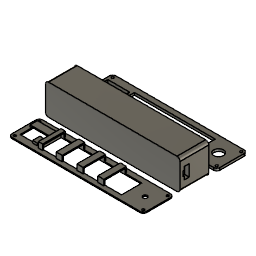
pomodoro (Autodesk Fusion 360 design; units mm, degrees)
Autodesk Fusion 360 part; units mm, degrees
sketch "Sketch1" plane through (0, 0, 0) normal (0, 0, 1) x (1, 0, 0)
  line L0 (66, 16.5) -> (-66, 16.5)
  line L1 (-66, 16.5) -> (-66, -16.5)
  line L2 (-66, -16.5) -> (66, -16.5)
  line L3 (66, -16.5) -> (66, 16.5)
  line L4 (66, 16.5) -> (-66, -16.5) construction
  line L5 (-66, 16.5) -> (66, -16.5) construction
  circle A0 centre (88, 0) radius 3.5
  line L6 (-74, 14) -> (-102, 14)
  line L7 (-102, 14) -> (-102, -14)
  line L8 (-102, -14) -> (-74, -14)
  line L9 (-74, -14) -> (-74, 14)
  line L10 (-74, 14) -> (-102, -14) construction
  line L11 (-102, 14) -> (-74, -14) construction
  line L12 (105, 25) -> (-105, 25)
  line L13 (-110, 20) -> (-110, -20)
  line L14 (-105, -25) -> (105, -25)
  line L15 (110, -20) -> (110, 20)
  line L16 (110, 25) -> (-110, -25) construction
  line L17 (-110, 25) -> (110, -25) construction
  circle A1 centre (88, 0) radius 8
  line L18 (-74, 9) -> (-102, 9)
  line L19 (-102, 9) -> (-102, -6)
  line L20 (-102, -6) -> (-74, -6)
  line L21 (-74, -6) -> (-74, 9)
  arc A2 (110, 20) -> (105, 25) centre (105, 20) ccw
  arc A3 (105, -25) -> (110, -20) centre (105, -20) ccw
  arc A4 (-110, -20) -> (-105, -25) centre (-105, -20) ccw
  arc A5 (-105, 25) -> (-110, 20) centre (-105, 20) ccw
  circle A6 centre (-105, -20) radius 2
  circle A7 centre (-105, 20) radius 2
  circle A8 centre (105, 20) radius 2
  circle A9 centre (105, -20) radius 2
  line L22 (-68, 18.5) -> (-61, 18.5)
  line L23 (-61, 18.5) -> (-61, -18.5)
  line L24 (-61, -18.5) -> (-68, -18.5)
  line L25 (-68, -18.5) -> (-68, 18.5)
  line L26 (-39, 18.5) -> (-29, 18.5)
  line L27 (-29, 18.5) -> (-29, -18.5)
  line L28 (-29, -18.5) -> (-39, -18.5)
  line L29 (-39, -18.5) -> (-39, 18.5)
  line L30 (-5, 18.5) -> (5, 18.5)
  line L31 (5, 18.5) -> (5, -18.5)
  line L32 (5, -18.5) -> (-5, -18.5)
  line L33 (-5, -18.5) -> (-5, 18.5)
  line L34 (0, 2.5) -> (0, 20)
  line L35 (39, 18.5) -> (29, 18.5)
  line L36 (29, 18.5) -> (29, -18.5)
  line L37 (29, -18.5) -> (39, -18.5)
  line L38 (39, -18.5) -> (39, 18.5)
  line L39 (-72, -16) -> (-104, -16)
  line L40 (-104, -16) -> (-104, -4)
  line L41 (-104, -4) -> (-72, -4)
  line L42 (-72, -4) -> (-72, -16)
  line L43 (-72, 16) -> (-80, 16)
  line L44 (-80, 16) -> (-80, 4)
  line L45 (-80, 4) -> (-72, 4)
  line L46 (-72, 4) -> (-72, 16)
  point P0 (-88, 0)
  dimension "d1" = 132
  dimension "d2" = 33
  dimension "d4" = 7
  dimension "d5" = 28
  dimension "d6" = 28
  dimension "d7" = 22
  dimension "d8" = 22
  dimension "d9" = 220
  dimension "d10" = 50
  dimension "d11" = 16
  dimension "d12" = 5
  dimension "d13" = 15
  dimension "d14" = 5
  dimension "d15" = 4
  dimension "d16" = 4
  dimension "d17" = 4
  dimension "d18" = 4
  dimension "d59" = 7
  dimension "d60" = 37
  dimension "d61" = 10
  dimension "d62" = 37
  dimension "d63" = 27
  dimension "d64" = 37
  dimension "d65" = 61
  constraint horizontal L0
  constraint perpendicular L0 L1
  constraint parallel L0 L2
  constraint parallel L1 L3
  constraint coincident L4 origin
  constraint coincident L5 origin
  constraint horizontal L6
  constraint perpendicular L6 L7
  constraint parallel L6 L8
  constraint parallel L7 L9
  constraint coincident L10 P0
  constraint coincident L11 P0
  constraint horizontal L12
  constraint perpendicular L12 L13
  constraint parallel L12 L14
  constraint parallel L13 L15
  constraint coincident L16 origin
  constraint coincident L17 origin
  constraint concentric A0 A1
  constraint horizontal L18
  constraint vertical L19
  constraint horizontal L20
  constraint vertical L21
  constraint coincident L7 L19.end
  constraint coincident L9 L18.start
  constraint coincident L16.start L12
  constraint coincident L16.start L15
  constraint tangent L12 A2
  constraint tangent L15 A2
  constraint coincident L17.end L15
  constraint coincident L17.end L14
  constraint tangent L15 A3
  constraint tangent L14 A3
  constraint equal A2 A3
  constraint coincident L16.end L13
  constraint coincident L16.end L14
  constraint tangent L13 A4
  constraint tangent L14 A4
  constraint equal A2 A4
  constraint coincident L17.start L12
  constraint coincident L17.start L13
  constraint tangent L12 A5
  constraint tangent L13 A5
  constraint equal A2 A5
  constraint concentric A4 A6
  constraint concentric A5 A7
  constraint concentric A2 A8
  constraint concentric A3 A9
  constraint horizontal L22
  constraint vertical L23
  constraint horizontal L24
  constraint vertical L25
  constraint horizontal L26
  constraint vertical L27
  constraint horizontal L28
  constraint vertical L29
  constraint horizontal L30
  constraint vertical L31
  constraint horizontal L32
  constraint vertical L33
  constraint symmetric L26.start L34 L35.start
  constraint symmetric L26.end L34 L35.end
  constraint symmetric L27.end L34 L36.end
  constraint symmetric L28.end L34 L37.end
  constraint horizontal L39
  constraint vertical L40
  constraint horizontal L41
  constraint vertical L42
  constraint horizontal L43
  constraint vertical L44
  constraint horizontal L45
  constraint vertical L46
  measures "d1" distance of L1.end L2.end
  measures "d2" distance of L0.end L1.end
  measures "d4" diameter of A0
  measures "d5" distance of L7.end L8.end
  measures "d6" distance of L6.end L7.end
  measures "d7" distance of L1 P0
  measures "d8" distance of L3 A0.centre
  measures "d9" distance of L16.end L17.end
  measures "d10" distance of L17.start L16.end
  measures "d11" diameter of A1
  measures "d12" distance of L6 L18
  measures "d13" distance of L18 L20
  measures "d14" radius of A2
  measures "d15" diameter of A6
  measures "d16" diameter of A7
  measures "d17" diameter of A8
  measures "d18" diameter of A9
  measures "d59" distance of L22.start L22.end
  measures "d60" distance of L22.start L24.end
  measures "d61" distance of L26.start L26.end
  measures "d62" distance of L26.start L28.end
  measures "d63" distance of L1 L29
  measures "d64" distance of L30.start L32.end
  measures "d65" distance of L1 L33
extrude "Extrude1" add sketch "Sketch1" along normal blind 4 contours L0 L35 L36 L38 | L2 L36 L37 L38 | L0 L30 L31 L34 | L0 L30 L33 L34 | L2 L31 L32 L33 | L0 L26 L27 L29 | L2 L27 L28 L29 | L0 L1 L2 L22 L23 L24 L25 | L6 L9 L18 L44 | L6 L9 L21 L43 L44 L45 L46 | L6 L7 L18 L44 | L7 L8 L9 L19 L21 L39 L40 L41 L42 | L7 L8 L9 L20 | L12 L13 L14 L15 A2 A3 A4 A5 makes body 1
extrude "Extrude2" add sketch "Sketch1" against normal blind 1.8 separate body contours L0 L35 L36 L38 | L2 L36 L37 L38 | L0 L30 L31 L34 | L0 L30 L33 L34 | L2 L31 L32 L33 | L0 L26 L27 L29 | L2 L27 L28 L29 | L0 L1 L2 L22 L23 L24 L25 | L6 L9 L21 L43 L44 L45 L46 | L7 L8 L9 L19 L21 L39 L40 L41 L42 | L12 L13 L14 L15 A2 A3 A4 A5 | A1 makes body 2
move_body "Move1" bodies 1 to x (1, 0, 0) y (0, 1, 0) z (0, 0, 1) at (0, 60, 0)
extrude "Extrude13" add sketch "Sketch1" against normal blind 11 contours L0 L2 L36 L38 | L0 L35 L36 L38 | L2 L36 L37 L38 | L0 L2 L31 L33 | L0 L30 L31 L34 | L0 L30 L33 L34 | L2 L31 L32 L33 | L0 L2 L27 L29 | L0 L26 L27 L29 | L2 L27 L28 L29 | L0 L1 L2 L23 | L0 L1 L2 L22 L23 L24 L25 bodies 2
extrude "Extrude14" cut sketch "Sketch1" against normal blind 9 contours L0 L2 L36 L38 | L0 L2 L31 L33 | L0 L2 L27 L29 | L0 L1 L2 L23 bodies 2
extrude "Extrude15" add sketch "Sketch1" against normal blind 5.5 contours L6 L9 L18 L44 | L6 L9 L21 L43 L44 L45 L46 | L9 L18 L21 L44 L45 | L7 L8 L9 L19 L21 L39 L40 L41 L42 | L7 L9 L19 L20 L21 L41 | L7 L8 L9 L20 bodies 2
extrude "Extrude16" cut sketch "Sketch1" against normal blind 3.5 contours L6 L9 L18 L44 | L9 L18 L21 L44 L45 | L7 L9 L19 L20 L21 L41 | L7 L8 L9 L20 bodies 2
move_body "Move2" bodies 2 to x (1, 0, 0) y (0, 1, 0) z (0, 0, 1) at (0, 0, 1.8)
chamfer "Chamfer1" distance 4 distance2 3 4 edges at (-88, 69, 4) (-102, 61.5, 4) (-88, 54, 4) (-74, 61.5, 4) measured on face at (105.3333, 60, 4) measured on face at (105.3333, 60, 4) measured on face at (105.3333, 60, 4) measured on face at (105.3333, 60, 4) on bodies 1
sketch "Sketch2" plane through (0, 0, 0) normal (0, 0, 1) x (1, 0, 0)
  line L0 (-105, 25) -> (105, 25)
  line L1 (110, 20) -> (110, -20)
  line L2 (105, -25) -> (-105, -25)
  line L3 (-110, -20) -> (-110, 20)
  arc A0 (-105, 25) -> (-110, 20) centre (-105, 20) ccw
  arc A1 (-110, -20) -> (-105, -25) centre (-105, -20) ccw
  arc A2 (105, -25) -> (110, -20) centre (105, -20) ccw
  arc A3 (110, 20) -> (105, 25) centre (105, 20) ccw
  line L4 (-102.5, 17.5) -> (102.5, 17.5)
  line L5 (102.5, 17.5) -> (102.5, -17.5)
  line L6 (102.5, -17.5) -> (-102.5, -17.5)
  line L7 (-102.5, -17.5) -> (-102.5, 17.5)
  line L8 (110, -10) -> (65, -10)
  line L9 (65, -10) -> (65, 10)
  line L10 (65, 10) -> (110, 10)
  line L11 (110, 10) -> (110, -10)
  line L12 (65, -10) -> (102.5, -10)
  line L13 (102.5, -10) -> (102.5, -12)
  line L14 (102.5, -12) -> (65, -12)
  line L15 (65, -12) -> (65, -10)
  line L16 (65, 10) -> (102.5, 10)
  line L17 (102.5, 10) -> (102.5, 12)
  line L18 (102.5, 12) -> (65, 12)
  line L19 (65, 12) -> (65, 10)
  line L20 (65, -12) -> (63, -12)
  line L21 (63, -12) -> (63, -7)
  line L22 (63, -7) -> (65, -7)
  line L23 (65, -7) -> (65, -12)
  line L24 (65, 12) -> (63, 12)
  line L25 (63, 12) -> (63, 7)
  line L26 (63, 7) -> (65, 7)
  line L27 (65, 7) -> (65, 12)
  circle A4 centre (105, 20) radius 1
  circle A5 centre (105, -20) radius 1
  circle A6 centre (-105, -20) radius 1
  circle A7 centre (-105, 20) radius 1
  line L28 (-68.5, 19) -> (-60.5, 19)
  line L29 (-60.5, 19) -> (-60.5, -19)
  line L30 (-60.5, -19) -> (-68.5, -19)
  line L31 (-68.5, -19) -> (-68.5, 19)
  line L32 (-39.5, 19) -> (-28.5, 19)
  line L33 (-28.5, 19) -> (-28.5, -19)
  line L34 (-28.5, -19) -> (-39.5, -19)
  line L35 (-39.5, -19) -> (-39.5, 19)
  line L36 (-5.5, -19) -> (5.5, -19)
  line L37 (5.5, -19) -> (5.5, 19)
  line L38 (5.5, 19) -> (-5.5, 19)
  line L39 (-5.5, 19) -> (-5.5, -19)
  line L40 (28.5, 19) -> (39.5, 19)
  line L41 (39.5, 19) -> (39.5, -19)
  line L42 (39.5, -19) -> (28.5, -19)
  line L43 (28.5, -19) -> (28.5, 19)
  line L44 (-102.5, -16.5) -> (-105, -16.5)
  line L45 (-105, -16.5) -> (-105, -3.5)
  line L46 (-105, -3.5) -> (-102.5, -3.5)
  line L47 (-102.5, -3.5) -> (-102.5, -16.5)
  dimension "d25" = 5
  dimension "d46" = 45
  dimension "d47" = 20
  dimension "d48" = 2
  dimension "d49" = 2
  dimension "d50" = 2
  constraint horizontal L0
  constraint vertical L1
  constraint horizontal L2
  constraint vertical L3
  constraint tangent L0 A0
  constraint tangent L3 A0
  constraint tangent L2 A1
  constraint tangent L3 A1
  constraint equal A0 A1
  constraint tangent L1 A2
  constraint tangent L2 A2
  constraint equal A0 A2
  constraint tangent L0 A3
  constraint tangent L1 A3
  constraint equal A0 A3
  constraint horizontal L4
  constraint vertical L5
  constraint horizontal L6
  constraint vertical L7
  constraint horizontal L8
  constraint vertical L9
  constraint horizontal L10
  constraint vertical L11
  constraint coincident L1 L8.start
  constraint horizontal L12
  constraint vertical L13
  constraint horizontal L14
  constraint vertical L15
  constraint horizontal L16
  constraint vertical L17
  constraint horizontal L18
  constraint vertical L19
  constraint horizontal L20
  constraint vertical L21
  constraint horizontal L22
  constraint vertical L23
  constraint horizontal L24
  constraint vertical L25
  constraint horizontal L26
  constraint vertical L27
  constraint concentric A3 A4
  constraint concentric A2 A5
  constraint concentric A1 A6
  constraint concentric A0 A7
  constraint horizontal L28
  constraint vertical L29
  constraint horizontal L30
  constraint vertical L31
  constraint horizontal L32
  constraint vertical L33
  constraint horizontal L34
  constraint vertical L35
  constraint horizontal L36
  constraint vertical L37
  constraint horizontal L38
  constraint vertical L39
  constraint horizontal L40
  constraint vertical L41
  constraint horizontal L42
  constraint vertical L43
  constraint horizontal L44
  constraint vertical L45
  constraint horizontal L46
  constraint vertical L47
  constraint coincident L7 L44.start
  measures "d25" radius of A0
  measures "d46" distance of L8.start L8.end
  measures "d47" distance of L8.start L10.end
  measures "d48" distance of L8.end L14.end
  measures "d49" distance of L9.end L18.end
  measures "d50" distance of L14.end L20.end
extrude "Extrude3" add sketch "Sketch2" along normal blind 40 separate body contours L0 L1 L2 L3 A0 A1 A2 A3 L4 L5 L6 L7 L8 L10 L13 L17 L28 L29 L30 L31 L32 L33 L34 L35 L36 L37 L38 L39 L40 L41 L42 L43 L44 L45 L46 | L1 L5 L8 L10 L11 makes body 3
extrude "Extrude17" add sketch "Sketch2" along normal blind 30.5 contours L4 L40 L41 L43 | L6 L41 L42 L43 | L4 L37 L38 L39 | L6 L36 L37 L39 | L4 L32 L33 L35 | L6 L33 L34 L35 | L4 L28 L29 L31 | L6 L29 L30 L31 | L7 L44 L45 L46 L47 bodies 3
extrude "Extrude12" add sketch "Sketch2" along normal blind 39 contours A4 | A5 | A6 | A7 bodies 3
chamfer "Chamfer2" distance 1 distance2 0.7 4 edges at (-105.9323, 20.3616, 39) (-105.9323, -19.6384, 39) (104.0677, -19.6384, 39) (104.0677, 20.3616, 39) measured on face at (-104.4163, 20.8119, 39.3333) measured on face at (-104.6815, -19.0521, 39.3333) measured on face at (105.4113, -19.0885, 39.6667) measured on face at (105.4113, 20.9115, 39.6667) on bodies 3
move_body "Move3" bodies 2 to x (1, 0, 0) y (0, -1, 0) z (0, 0, -1) at (0, -60, 1.8)
extrude "Extrude4" add sketch "Sketch2" against normal blind 5 contours L0 L1 L2 L3 A0 A1 A2 A3 L4 L5 L6 L7 L8 L10 L13 L17 L28 L29 L30 L31 L32 L33 L34 L35 L36 L37 L38 L39 L40 L41 L42 L43 L44 L45 L46 | L1 L5 L8 L10 L11 | L5 L10 L16 L17 L18 L19 L27 | L5 L8 L9 L10 L12 L16 L23 L27 | L5 L8 L12 L13 L14 L15 L23 | L4 L5 L6 L9 L14 L18 L20 L21 L22 L24 L25 L26 L41 | L9 L19 L24 L25 L26 L27 | L9 L15 L20 L21 L22 L23 | L4 L6 L41 L43 | L4 L40 L41 L43 | L6 L41 L42 L43 | L4 L6 L37 L43 | L4 L6 L37 L39 | L4 L37 L38 L39 | L6 L36 L37 L39 | L4 L6 L33 L39 | L4 L6 L33 L35 | L4 L32 L33 L35 | L6 L33 L34 L35 | L4 L6 L29 L35 | L4 L6 L29 L31 | L4 L28 L29 L31 | L6 L29 L30 L31 | L4 L6 L7 L31 L47 | L7 L44 L45 L46 L47 | A4 | A5 | A6 | A7 bodies 3
sketch "Sketch3" plane through (110, 0, 0) normal (1, 0, 0) x (0, 1, 0)
  line L0 (20, -5) -> (20, 40)
  line L1 (20, 40) -> (-20, 40)
  line L2 (-20, 40) -> (-20, -5)
  line L3 (-20, -5) -> (20, -5)
  line L4 (-9.5, 0) -> (-9.5, 8)
  line L5 (-9.5, 8) -> (9.5, 8)
  line L6 (9.5, 8) -> (9.5, 0)
  line L7 (9.5, 0) -> (-9.5, 0)
  line L8 (4, -2) -> (-4, -2)
  line L9 (-4, -2) -> (-4, 2)
  line L10 (-4, 2) -> (4, 2)
  line L11 (4, 2) -> (4, -2)
  line L12 (4, -2) -> (-4, 2) construction
  line L13 (-4, -2) -> (4, 2) construction
  dimension "d32" = 19
  dimension "d33" = 8
  constraint vertical L4
  constraint horizontal L5
  constraint vertical L6
  constraint perpendicular L4 L7
  constraint horizontal L8
  constraint perpendicular L8 L9
  constraint parallel L8 L10
  constraint parallel L9 L11
  constraint coincident L12 origin
  constraint coincident L13 origin
  measures "d32" distance of L6.end L4.start
  measures "d33" distance of L6.end L5.end
extrude "Extrude5" cut sketch "Sketch3" against normal blind 10 contours L4 L5 L6 L7 L9 L10 L11 | L7 L9 L10 L11 | L7 L8 L9 L11 bodies 3
extrude "Extrude6" add 1 faces at (35, -8.3333, -5) along direction (0, 0, -1) blind 1 on bodies 3 bodies 3
sketch "Sketch4" plane through (0, 25, 0) normal (0, 1, 0) x (-1, 0, 0)
  line L0 (105, -6) -> (105, 40)
  line L1 (105, 40) -> (-105, 40)
  line L2 (-105, 40) -> (-105, -6)
  line L3 (-105, -6) -> (105, -6)
  circle A0 centre (0, 20) radius 6.5
  circle A1 centre (0, 20) radius 8
  line L4 (-4.958, 15.7966) -> (-6.8067, 15.7966)
  line L5 (-4.9612, 24.1996) -> (-6.8091, 24.1996)
  line L6 (4.9605, 24.2004) -> (6.8086, 24.2004)
  line L7 (4.9573, 15.7958) -> (6.8062, 15.7958)
  line L8 (4.9605, 24.2004) -> (-4.9612, 24.1996)
  line L9 (4.9573, 15.7958) -> (-4.958, 15.7966)
  dimension "d38" = 13
  dimension "d41" = 16
  constraint concentric A0 A1
  constraint coincident A0 L4.start
  constraint coincident A1 L4.end
  constraint horizontal L4
  constraint coincident A0 L5.start
  constraint coincident A1 L5.end
  constraint parallel L4 L5
  constraint coincident A0 L6.start
  constraint coincident A1 L6.end
  constraint parallel L5 L6
  constraint coincident A0 L7.start
  constraint coincident A1 L7.end
  constraint parallel L6 L7
  measures "d38" diameter of A0
  measures "d41" diameter of A1
extrude "Extrude7" cut sketch "Sketch4" against normal blind 15 contours A0 L8 L9 | A0 L8 | A0 L9 bodies 3
extrude "Extrude8" add sketch "Sketch4" against normal blind 12 contours A0 L8 | A0 A1 L5 L6 | A0 A1 L4 L7 | A0 L9 bodies 3
extrude "Extrude9" cut sketch "Sketch4" against normal blind 10 contours A0 L8 | A0 L9 bodies 3
extrude "Extrude10" add sketch "Sketch2" along normal blind 2 contours L5 L10 L16 L17 L18 L19 L27 | L5 L8 L12 L13 L14 L15 L23 | L9 L19 L24 L25 L26 L27 | L9 L15 L20 L21 L22 L23 bodies 3
extrude "Extrude11" add 1 faces at (35, -8.3333, -6) along direction (0, 0, -1) blind 1 on bodies 3 bodies 3
move_body "Move4" bodies 3 to x (1, 0, 0) y (0, 0, -1) z (0, 1, 0) at (0, -18, 25)
